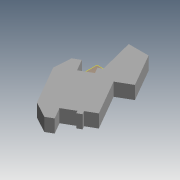
# Autodesk Inventor part: Part2
Saved by Autodesk Inventor 2014 SP1 (Build 180222100, 222)
## iProperties
Created: 2014-04-03
Part Number: Part2
Material: Generic
Document SubType Name: Modeling
Designer: tom
Density: 1 g/cm^3
Appearance: Default
Author: tom
Autodesk Inventor part; units mm, degrees
ref_plane "YZ Plane" through (0, 0, 0) normal (1, 0, 0) x (0, 1, 0)
ref_plane "XZ Plane" through (0, 0, 0) normal (0, 1, 0) x (-1, 0, 0)
ref_plane "XY Plane" through (0, 0, 0) normal (0, 0, 1) x (1, 0, 0)
ref_plane "Work Plane3" through (-98.2192, 25.6748, -72.651) normal (0, 1, 0) x (1, 0, 0)
sketch "Sketch1" plane through (-98.2192, 25.6748, -72.651) normal (0, 1, 0) x (1, 0, 0)
  line L0 (108.2722, -112.7231) -> (109.1382, -112.2231) construction
  line L1 (108.6382, -111.3571) -> (109.1382, -112.2231) construction
  line L2 (101.5917, -99.1522) -> (114.8917, -122.1885)
  line L3 (114.8917, -122.1885) -> (108.6563, -125.7885)
  line L4 (108.6563, -125.7885) -> (109.9613, -128.0488)
  line L5 (109.9613, -128.0488) -> (107.3632, -129.5488)
  line L6 (107.3632, -129.5488) -> (106.3632, -127.8168)
  line L7 (106.3632, -127.8168) -> (98.8635, -132.1468)
  line L8 (98.8635, -132.1468) -> (103.1935, -139.6466)
  line L9 (79.4712, -121.2385) -> (82.4842, -126.4571) construction
  line L10 (103.1935, -139.6466) -> (98.8633, -142.1466)
  line L11 (83.0235, -104.7111) -> (90.5232, -100.3811)
  line L12 (90.5232, -100.3811) -> (88.3182, -96.5619)
  line L13 (88.3182, -96.5619) -> (90.8427, -95.1044)
  line L14 (83.0235, -104.7111) -> (78.6935, -97.2113)
  line L15 (73.6327, -111.1259) -> (88.2377, -136.4225)
  line L16 (78.6935, -97.2113) -> (74.3633, -99.7113)
  line L17 (90.8427, -95.1044) -> (85.0892, -72.651)
  line L18 (104.7842, -84.0219) -> (98.2192, -72.651)
  line L19 (98.2192, -72.651) -> (85.0892, -72.651)
  line L20 (88.2377, -136.4225) -> (98.8633, -142.1466)
  line L21 (74.3633, -99.7113) -> (73.6327, -111.1259)
  line L22 (98.2192, -72.651) -> (104.7842, -84.0219)
  line L23 (104.7842, -84.0219) -> (101.5917, -99.1522)
  dimension "d1" = 26.6
  dimension "d4" = 7.2
  dimension "d5" = 2.61
  dimension "d6" = 3
  dimension "d7" = 2
  dimension "d8" = 8.66
  dimension "d9" = 8.66
  dimension "d10" = 5
  dimension "d11" = 8.66
  dimension "d12" = 31.68
  dimension "d13" = 4.41
  dimension "d14" = 2.915
  dimension "d17" = 8.66
  dimension "d18" = 29.21
  dimension "d20" = 10.27
  dimension "d21" = 5
  dimension "d22" = 23.1789
  dimension "d23" = 13.13
  dimension "d31" = 13.13
  constraints: 48 end point, 7 perpendicular, 1 collinear, 1 parallel
  measures "d1" distance of L2.start L2.end
  measures "d4" distance of L2.end L3.end
  measures "d5" distance of L3.end L4.end
  measures "d6" distance of L4.end L5.end
  measures "d7" distance of L5.end L6.end
  measures "d8" distance of L6.end L7.end
  measures "d9" distance of L7.end L8.end
  measures "d10" distance of L8.end L10.end
  measures "d11" distance of L11.start L11.end
  measures "d12" distance between parallel lines of L7 L11
  measures "d13" distance of L11.end L12.end
  measures "d14" distance of L12.end L13.end
  measures "d17" distance of L11.start L14.end
  measures "d18" distance of L15.start L15.end
  measures "d20" distance from line of L10 L15.end
  measures "d21" distance of L14.end L16.end
  measures "d22" distance of L13.end L17.end
  measures "d23" distance of L18.end L17.end
  measures "d31" distance of L18.start L18.end
extrude "Extrusion1" add sketch "Sketch1" along normal blind 8.66
pattern_circular "Circular Pattern2" count 3 over 360 about axis through (0, 25.6748, 0) along (0, 1, 0) of "Extrusion1"
sketch "Sketch2" plane through (-98.2192, 34.3348, -72.651) normal (0, 1, 0) x (1, 0, 0)
  line L0 (101.5917, -99.1522) -> (104.7842, -84.0219) projected
  line L1 (104.7842, -84.0219) -> (121.3528, -67.8125) projected
  line L2 (121.3528, -67.8125) -> (123.8772, -69.27) projected
  line L3 (123.8772, -69.27) -> (126.0822, -65.4508) projected
  line L4 (126.0822, -65.4508) -> (133.582, -69.7808) projected
  line L5 (133.582, -69.7808) -> (129.252, -77.2806) projected
  line L6 (129.252, -77.2806) -> (133.5821, -79.7806) projected
  line L7 (133.5821, -79.7806) -> (143.8327, -74.706) projected
  line L8 (143.8327, -74.706) -> (158.4377, -49.4094) projected
  line L9 (158.4377, -49.4094) -> (158.0821, -37.3454) projected
  line L10 (158.0821, -37.3454) -> (153.752, -34.8454) projected
  line L11 (153.752, -34.8454) -> (149.422, -42.3451) projected
  line L12 (149.422, -42.3451) -> (141.9222, -38.0151) projected
  line L13 (141.9222, -38.0151) -> (142.9222, -36.2831) projected
  line L14 (142.9222, -36.2831) -> (140.3242, -34.7831) projected
  line L15 (140.3242, -34.7831) -> (139.0192, -37.0434) projected
  line L16 (139.0192, -37.0434) -> (132.7838, -33.4434) projected
  line L17 (132.7838, -33.4434) -> (119.4838, -56.4797) projected
  line L18 (119.4838, -56.4797) -> (104.7842, -61.28) projected
  line L19 (104.7842, -61.28) -> (82.4622, -55.036) projected
  line L20 (82.4622, -55.036) -> (82.4622, -52.121) projected
  line L21 (82.4622, -52.121) -> (78.0522, -52.121) projected
  line L22 (78.0522, -52.121) -> (78.0522, -43.461) projected
  line L23 (78.0522, -43.461) -> (86.7122, -43.461) projected
  line L24 (86.7122, -43.461) -> (86.7122, -38.461) projected
  line L25 (86.7122, -38.461) -> (77.1922, -32.121) projected
  line L26 (77.1922, -32.121) -> (47.9822, -32.121) projected
  line L27 (47.9822, -32.121) -> (37.7122, -38.461) projected
  line L28 (37.7122, -38.461) -> (37.7122, -43.461) projected
  line L29 (37.7122, -43.461) -> (46.3722, -43.461) projected
  line L30 (46.3722, -43.461) -> (46.3722, -52.121) projected
  line L31 (46.3722, -52.121) -> (44.3722, -52.121) projected
  line L32 (44.3722, -52.121) -> (44.3722, -55.121) projected
  line L33 (44.3722, -55.121) -> (46.9822, -55.121) projected
  line L34 (46.9822, -55.121) -> (46.9822, -62.321) projected
  line L35 (46.9822, -62.321) -> (73.5822, -62.321) projected
  line L36 (73.5822, -62.321) -> (85.0892, -72.651) projected
  line L37 (85.0892, -72.651) -> (90.8427, -95.1044) projected
  line L38 (90.8427, -95.1044) -> (88.3182, -96.5619) projected
  line L39 (88.3182, -96.5619) -> (90.5232, -100.3811) projected
  line L40 (90.5232, -100.3811) -> (83.0235, -104.7111) projected
  line L41 (83.0235, -104.7111) -> (78.6935, -97.2113) projected
  line L42 (78.6935, -97.2113) -> (74.3633, -99.7113) projected
  line L43 (74.3633, -99.7113) -> (73.6327, -111.1259) projected
  line L44 (73.6327, -111.1259) -> (88.2377, -136.4225) projected
  line L45 (88.2377, -136.4225) -> (98.8633, -142.1466) projected
  line L46 (98.8633, -142.1466) -> (103.1935, -139.6466) projected
  line L47 (103.1935, -139.6466) -> (98.8635, -132.1468) projected
  line L48 (98.8635, -132.1468) -> (106.3632, -127.8168) projected
  line L49 (106.3632, -127.8168) -> (107.3632, -129.5488) projected
  line L50 (107.3632, -129.5488) -> (109.9613, -128.0488) projected
  line L51 (109.9613, -128.0488) -> (108.6563, -125.7885) projected
  line L52 (108.6563, -125.7885) -> (114.8917, -122.1885) projected
  line L53 (114.8917, -122.1885) -> (101.5917, -99.1522) projected
  circle A0 centre (98.2192, -72.651) radius 1.5
  line L54 (98.2192, -72.651) -> (104.7842, -84.0219) construction
  line L55 (98.2192, -72.651) -> (85.0892, -72.651) construction
  line L56 (98.2192, -72.651) -> (104.7842, -61.28) construction
  dimension "d35" = 3
  constraints: 6 end point, 2 parallel, 1 centre point, 1 coincident
  measures "d35" diameter of A0
body "Solid1"
